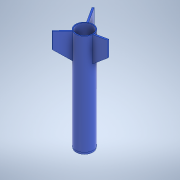
# Autodesk Inventor part: tail
Saved by Autodesk Inventor 2020 (Build 240168000, 168)
## iProperties
Created: 2021-01-23
Part Number: tail
Material: ABS Plastic
Document SubType Name: Modeling
Designer: 0x6f736f646f
Density: 1.06 g/cm^3
Appearance: Smooth - White
Author: 0x6f736f646f
Autodesk Inventor part; units mm, degrees
ref_plane "YZ Plane" through (0, 0, 0) normal (1, 0, 0) x (0, 1, 0)
ref_plane "XZ Plane" through (0, 0, 0) normal (0, 1, 0) x (-1, 0, 0)
ref_plane "XY Plane" through (0, 0, 0) normal (0, 0, 1) x (1, 0, 0)
sketch "Sketch1" plane through (0, 0, 0) normal (0, 1, 0) x (-1, 0, 0)
  circle A0 centre (0, 0) radius 15
  circle A1 centre (0, 0) radius 15.9
  circle A2 centre (0, 0) radius 16.8
  dimension "d0" = 30
  dimension "d1" = 31.8
  dimension "d2" = 33.6
  constraints: 3 centre point, 3 coincident
  measures "d0" diameter of A0
  measures "d1" diameter of A1
  measures "d2" diameter of A2
extrude "Extrusion1" add sketch "Sketch1" along normal blind 96 and the other way blind 100 contours A1
extrude "Extrusion2" add sketch "Sketch1" along normal blind 96 and the other way blind 96 contours A2
sketch "Sketch4" plane through (0, 0, 0) normal (0, 0, 1) x (1, 0, 0)
  line L0 (45, 99.9302) -> (45, 71.173)
  line L1 (45, 71.173) -> (15, 46)
  line L2 (15, 46) -> (15, 96)
  line L3 (15, 96) -> (45, 101.173)
  line L4 (45, 101.173) -> (45, 99.9302)
  line L5 (-15, 96) -> (15, 96) projected
  line L6 (16.8, 96) -> (-16.8, 96) projected
  line L7 (-15, 96) -> (15, 96) projected
  line L8 (15.9, -100) -> (15, -100) projected
  line L9 (15, -100) -> (15, 96) projected
  line L10 (15, 96) -> (16.8, 96) projected
  line L11 (16.8, 96) -> (16.8, -96) projected
  line L12 (16.8, -96) -> (15.9, -96) projected
  line L13 (-15, -100) -> (-15.9, -100) projected
  line L14 (-16.8, -96) -> (-16.8, 96) projected
  line L15 (-16.8, 96) -> (-15, 96) projected
  line L16 (-15, 96) -> (-15, -100) projected
  line L17 (-15.9, -96) -> (-16.8, -96) projected
  line L18 (15.9, -96) -> (15.9, -100) projected
  line L19 (-15.9, -100) -> (-15.9, -96) projected
  point P0 (0, 0)
  point P1 (16.8, 47.5104)
  dimension "d18" = 50
  dimension "d21" = 50
  dimension "d24" = 30
  dimension "d25" = 30
  constraints: 10 end point, 2 vertical, 1 coincident, 1 parallel, 1 point on line
  measures "d18" distance of L2.end L1.end
  measures "d21" angle of L2 L1
  measures "d24" distance of L3.end L0.end
  measures "d25" distance between parallel lines of L9 L0
extrude "Extrusion4" add sketch "Sketch4" along normal mid plane 3 contours L0 L1 L11 L6 L3 L4
pattern_circular "Circular Pattern2" count 3 over 360 about axis through (0, -10, 0) along (0, 1, 0) of "Extrusion4"
body "Solid1"
